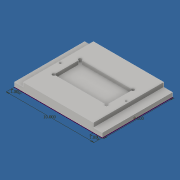
# Autodesk Inventor part: Case Jig
Saved by Autodesk Inventor 2,016 (Build 200138000, 138)
## iProperties
Created: 2015-09-01
Part Number: Case Jig
Material: Generic
Document SubType Name: Modeling
Designer: Sam Clay
Density: 1 g/cm^3
Appearance: Default
Author: Sam Clay
Autodesk Inventor part; units mm, degrees
ref_plane "YZ Plane" through (0, 0, 0) normal (1, 0, 0) x (0, 1, 0)
ref_plane "XZ Plane" through (0, 0, 0) normal (0, 1, 0) x (-1, 0, 0)
ref_plane "XY Plane" through (0, 0, 0) normal (0, 0, 1) x (1, 0, 0)
sketch "Sketch1" plane through (0, 0, 0) normal (0, 1, 0) x (-1, 0, 0)
  line L0 (127, 101.6) -> (101.6, 101.6)
  line L1 (-127, 101.6) -> (-127, -101.6)
  line L2 (-127, -101.6) -> (-101.6, -101.6)
  line L3 (127, -101.6) -> (127, 101.6)
  line L4 (127, 101.6) -> (-127, -101.6) construction
  line L5 (-127, 101.6) -> (127, -101.6) construction
  line L6 (127, -101.6) -> (101.6, -101.6)
  line L7 (101.6, -101.6) -> (101.6, 101.6)
  line L8 (101.6, 101.6) -> (127, 101.6)
  line L9 (127, 101.6) -> (127, -101.6)
  line L10 (-127, -101.6) -> (-101.6, -101.6)
  line L11 (-101.6, -101.6) -> (-101.6, 101.6)
  line L12 (-101.6, 101.6) -> (-127, 101.6)
  line L13 (-127, 101.6) -> (-127, -101.6)
  line L14 (101.6, -101.6) -> (127, -101.6)
  line L15 (101.6, 101.6) -> (-101.6, 101.6)
  line L16 (-101.6, 101.6) -> (-127, 101.6)
  line L17 (-101.6, -101.6) -> (101.6, -101.6)
  point P0 (0, 0)
  dimension "d0" = 254
  dimension "d1" = 203.2
  dimension "d2" = 25.4
  dimension "d3" = 25.4
  constraints: 36 end point, 14 parallel, 5 horizontal, 5 perpendicular, 2 midpoint, 1 point on line
  measures "d0" distance of L0.start L1.start
  measures "d1" distance of L1.end L1.start
  measures "d2" distance of L0.end L8.end
  measures "d3" distance of L12.end L11.end
extrude "Extrusion1" add sketch "Sketch1" along normal blind 25.4 contours L7 L17 L11 L15
extrude "Extrusion2" add sketch "Sketch1" along normal blind 12.7 contours L3 L6 L7 L0 | L11 L2 L1 L12
sketch "Sketch2" plane through (0, 25.4, 0) normal (0, 1, 0) x (1, 0, 0)
  line L0 (-76.2, -38.1) -> (76.2, -38.1)
  line L1 (76.2, -38.1) -> (76.2, 38.1)
  line L2 (76.2, 38.1) -> (-76.2, 38.1)
  line L3 (-76.2, 38.1) -> (-76.2, -38.1)
  line L4 (-76.2, -38.1) -> (76.2, 38.1) construction
  line L5 (76.2, -38.1) -> (-76.2, 38.1) construction
  circle A0 centre (-76.2, 38.1) radius 4.7625
  circle A1 centre (76.2, 38.1) radius 4.7625
  circle A2 centre (76.2, -38.1) radius 4.7625
  circle A3 centre (-76.2, -38.1) radius 4.7625
  point P0 (0, 0)
  dimension "d8" = 152.4
  dimension "d9" = 76.2
  dimension "d10" = 9.525
  dimension "d11" = 9.525
  dimension "d12" = 9.525
  dimension "d13" = 9.525
  constraints: 12 end point, 4 centre point, 4 coincident, 2 midpoint, 2 parallel, 1 horizontal, 1 perpendicular
  measures "d8" distance of L0.start L0.end
  measures "d9" distance of L1.end L0.end
  measures "d10" diameter of A0
  measures "d11" diameter of A1
  measures "d12" diameter of A2
  measures "d13" diameter of A3
extrude "Extrusion3" cut sketch "Sketch2" against normal blind 11.43
sketch "Sketch3" plane through (0, 25.4, 0) normal (0, 1, 0) x (1, 0, 0)
  circle A0 centre (-95.25, 0) radius 3.175
  line L0 (-76.2, -33.3375) -> (-76.2, 33.3375) projected
  point P0 (0, 0)
  dimension "d16" = 6.35
  dimension "d17" = 19.05
  constraints: 1 centre point
  measures "d16" diameter of A0
  measures "d17" distance from line of A0.centre L0
extrude "Extrusion4" cut sketch "Sketch3" against normal blind 12.7
mirror "Mirror1" about plane through (0, 0, 0) normal (1, 0, 0) of "Extrusion4"
equation "\"d11\" = d10"
equation "\"d12\" = d10"
equation "\"d13\" = d10"
body "Solid1"
